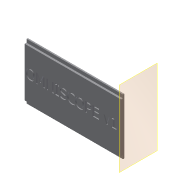
# Autodesk Inventor part: 01_Camera_Module_Lit
Saved by Autodesk Inventor 2019.4 (Build 234330000, 330)
## iProperties
Created: 2021-09-23
Part Number: 01_Camera_Module_Lit
Material: Generisch
Document SubType Name: Modeling
Designer: Muriel
Density: 1 g/cm^3
Appearance: Vorgabe
Mass: 2.33527 g
Surface Area: 32.2894 cm^2
Volume: 2.33527 cm^3
Author: Muriel
Autodesk Inventor part; units mm, degrees
ref_plane "YZ Plane" through (0, 0, 0) normal (1, 0, 0) x (0, 1, 0)
ref_plane "Arbeitsebene1" through (50, 3.7048, -4.525) normal (1, 0, 0) x (0, 0, -1)
sketch "Skizze1" plane through (50, 3.7048, -4.525) normal (1, 0, 0) x (0, 0, -1)
  line L0 (12.625, 1.4952) -> (9.775, 1.4952) projected
  line L1 (8.775, -0.2048) -> (8.475, -0.2048) projected
  line L2 (-3.525, -3.7048) -> (12.275, -3.7048) projected
  line L3 (13.275, -2.7048) -> (12.275, -3.7048) projected
  circle A0 centre (10.275, -2.1048) radius 0.95 projected
  circle A1 centre (-1.525, -2.1048) radius 0.95 projected
  line L4 (-2.525, 29.0952) -> (-2.525, 27.8724) projected
  line L5 (-1.025, 27.8724) -> (-2.525, 27.8724) projected
  line L6 (-1.025, 28.0952) -> (-1.025, 27.8724) projected
  line L7 (-0.025, 29.0952) -> (-1.025, 28.0952) projected
  line L8 (-0.025, 29.0952) -> (-2.525, 29.0952) projected
  line L9 (-4.525, 26.8952) -> (-2.825, 26.8952)
  line L10 (-2.825, 26.8952) -> (-2.825, 1.4952)
  line L11 (-2.825, 1.4952) -> (-4.525, 1.4952)
  line L12 (-4.525, 1.4952) -> (-4.525, 26.8952)
  line L13 (-2.825, 26.8952) -> (-3.525, 26.8952)
  line L14 (-3.525, 26.8952) -> (-3.525, 28.5952)
  line L15 (-3.525, 28.5952) -> (-2.825, 28.5952)
  line L16 (-2.825, 28.5952) -> (-2.825, 26.8952)
  line L17 (-2.825, 1.4952) -> (-3.525, 1.4952)
  line L18 (-3.525, 1.4952) -> (-3.525, -0.4048)
  line L19 (-3.525, -0.4048) -> (-2.825, -0.4048)
  line L20 (-2.825, -0.4048) -> (-2.825, 1.4952)
  line L21 (8.775, 28.5952) -> (8.475, 28.5952) projected
  line L22 (9.775, 26.8952) -> (9.775, 27.5952) projected
  line L23 (12.625, 26.8952) -> (9.775, 26.8952) projected
  line L24 (12.625, 1.4952) -> (12.625, 26.8952) projected
  line L25 (9.775, 1.4952) -> (9.775, 0.7952) projected
  line L26 (8.775, -0.2048) -> (9.775, 0.7952) projected
  line L27 (-3.525, -3.7048) -> (-4.525, -2.7048) projected
  line L28 (13.275, -2.7048) -> (13.275, 31.0952) projected
  line L29 (12.275, 32.0952) -> (13.275, 31.0952) projected
  line L30 (-3.525, 32.0952) -> (12.275, 32.0952) projected
  line L31 (-4.525, 31.0952) -> (-3.525, 32.0952) projected
  circle A2 centre (10.275, 30.4952) radius 0.95 projected
  circle A3 centre (-1.525, 30.4952) radius 0.95 projected
  line L32 (-3.6948, -0.7048) -> (-3.6948, 1.2952) projected
  line L33 (-4.525, 1.2952) -> (-4.525, -2.7048) projected
  line L34 (-4.525, 27.0952) -> (-4.525, 31.0952) projected
  line L35 (-3.6948, 27.0952) -> (-3.6948, 29.0952) projected
  line L36 (9.775, 27.5952) -> (8.775, 28.5952) projected
  line L37 (8.475, 29.0952) -> (8.475, 28.5952) projected
  line L38 (8.475, -0.2048) -> (8.475, -0.7048) projected
  line L39 (8.475, -0.7048) -> (-1.425, -0.7048) projected
  line L40 (-3.6948, 29.0952) -> (-2.425, 29.0952) projected
  line L41 (-1.425, 29.0952) -> (8.475, 29.0952) projected
  line L42 (-1.425, -0.7048) -> (-1.425, 0.2952) projected
  line L43 (-1.425, 0.2952) -> (-2.425, 0.2952) projected
  line L44 (-2.425, 0.2952) -> (-2.425, -0.7048) projected
  line L45 (-2.425, -0.7048) -> (-3.6948, -0.7048) projected
  line L46 (-3.6948, 1.2952) -> (-4.525, 1.2952) projected
  line L47 (-4.525, 27.0952) -> (-3.6948, 27.0952) projected
  line L48 (-2.425, 29.0952) -> (-2.425, 28.0952) projected
  line L49 (-2.425, 28.0952) -> (-1.425, 28.0952) projected
  line L50 (-1.425, 28.0952) -> (-1.425, 29.0952) projected
  point P0 (-4.525, -3.7048)
  point P1 (-3.525, 29.0952)
  point P2 (12.675, 25.9097)
  point P3 (12.675, 0.5181)
  point P4 (-4.525, -0.7048)
  point P5 (-4.525, 29.0952)
  point P6 (-1.525, -0.7048)
  point P7 (-2.525, 28.0952)
  point P8 (-1.525, 28.0952)
  point P9 (-1.525, 29.0952)
  point P10 (-2.525, -0.7048)
  constraints: 24 end point, 6 parallel, 3 horizontal, 3 perpendicular, 2 other
ref_plane "Arbeitsebene2" through (0, 5.25, -6.015) normal (-1, 0, 0) x (0, 0, 1)
ref_plane "Work Plane3" through (0, 1.51, -17.96) normal (1, 0, 0) x (0, 1, 0)
extrude "Extrusion1" add sketch "Skizze1" against normal up to surface (50 mm away) contours L9 L10 L11 L12 | L14 L15 L16 L9 | L11 L20 L19 L18
sketch "Skizze3" plane through (50, 5.2, 0) normal (0, 0, 1) x (1, 0, 0)
  line L0 (-49.4037, 15.6382) -> (-1.8416, 15.6382) construction
  line L1 (-1.8416, 15.6382) -> (-1.8416, 10.3786) construction
  line L2 (-1.8416, 10.3786) -> (-49.4037, 10.3786) construction
  line L3 (-49.4037, 10.3786) -> (-49.4037, 15.6382) construction
  spline S0 degree 2 poles (-45.3219, 14.9552) (-45.0356, 14.6198) (-44.7166, 13.6383) (-44.7166, 13.0084) knots 0 0 0 1 2 2 2
  spline S1 degree 2 poles (-44.7166, 13.0084) (-44.7166, 12.3949) (-45.0274, 11.4011) (-45.3219, 11.0657) knots 0 0 0 1 2 2 2
  spline S2 degree 2 poles (-45.3219, 11.0657) (-45.6327, 10.7139) (-46.4548, 10.3786) (-46.9497, 10.3786) knots 0 0 0 1 2 2 2
  spline S3 degree 2 poles (-46.9497, 10.3786) (-47.4609, 10.3786) (-48.2789, 10.7262) (-48.5775, 11.0657) knots 0 0 0 1 2 2 2
  spline S4 degree 2 poles (-48.5775, 11.0657) (-48.8679, 11.4011) (-49.1787, 12.3867) (-49.1787, 13.0084) knots 0 0 0 1 2 2 2
  spline S5 degree 2 poles (-49.1787, 13.0084) (-49.1787, 13.6423) (-48.8638, 14.6076) (-48.5734, 14.9552) knots 0 0 0 1 2 2 2
  spline S6 degree 2 poles (-48.5734, 14.9552) (-48.2789, 15.2906) (-47.4569, 15.6382) (-46.9497, 15.6382) knots 0 0 0 1 2 2 2
  spline S7 degree 2 poles (-46.9497, 15.6382) (-46.4344, 15.6382) (-45.6082, 15.2783) (-45.3219, 14.9552) knots 0 0 0 1 2 2 2
  spline S8 degree 2 poles (-45.416, 13.0084) (-45.416, 13.5074) (-45.6327, 14.2804) (-45.829, 14.534) knots 0 0 0 1 2 2 2
  spline S9 degree 2 poles (-45.829, 14.534) (-46.0295, 14.7957) (-46.5939, 15.0575) (-46.9456, 15.0575) knots 0 0 0 1 2 2 2
  spline S10 degree 2 poles (-46.9456, 15.0575) (-47.3096, 15.0575) (-47.8577, 14.8039) (-48.0663, 14.534) knots 0 0 0 1 2 2 2
  spline S11 degree 2 poles (-48.0663, 14.534) (-48.2667, 14.2763) (-48.4793, 13.4992) (-48.4793, 13.0084) knots 0 0 0 1 2 2 2
  spline S12 degree 2 poles (-48.4793, 13.0084) (-48.4793, 12.0145) (-47.645, 10.9593) (-46.9456, 10.9593) knots 0 0 0 1 2 2 2
  spline S13 degree 2 poles (-46.9456, 10.9593) (-46.2462, 10.9593) (-45.416, 12.0145) (-45.416, 13.0084) knots 0 0 0 1 2 2 2
  line L4 (-39.6532, 10.4849) -> (-40.324, 10.4849)
  line L5 (-40.324, 10.4849) -> (-40.324, 14.8325)
  line L6 (-40.324, 14.8325) -> (-41.6409, 11.8755)
  line L7 (-41.6409, 11.8755) -> (-42.0499, 11.8755)
  line L8 (-42.0499, 11.8755) -> (-43.3546, 14.8325)
  line L9 (-43.3546, 14.8325) -> (-43.3546, 10.4849)
  line L10 (-43.3546, 10.4849) -> (-43.9804, 10.4849)
  line L11 (-43.9804, 10.4849) -> (-43.9804, 15.5319)
  line L12 (-43.9804, 15.5319) -> (-43.0642, 15.5319)
  line L13 (-43.0642, 15.5319) -> (-41.8045, 12.7221)
  line L14 (-41.8045, 12.7221) -> (-40.5857, 15.5319)
  line L15 (-40.5857, 15.5319) -> (-39.6532, 15.5319)
  line L16 (-39.6532, 15.5319) -> (-39.6532, 10.4849)
  line L17 (-35.0193, 10.4849) -> (-35.7719, 10.4849)
  line L18 (-35.7719, 10.4849) -> (-38.005, 14.8366)
  line L19 (-38.005, 14.8366) -> (-38.005, 10.4849)
  line L20 (-38.005, 10.4849) -> (-38.6307, 10.4849)
  line L21 (-38.6307, 10.4849) -> (-38.6307, 15.5319)
  line L22 (-38.6307, 15.5319) -> (-37.6778, 15.5319)
  line L23 (-37.6778, 15.5319) -> (-35.6451, 11.536)
  line L24 (-35.6451, 11.536) -> (-35.6451, 15.5319)
  line L25 (-35.6451, 15.5319) -> (-35.0193, 15.5319)
  line L26 (-35.0193, 15.5319) -> (-35.0193, 10.4849)
  line L27 (-32.2381, 10.4849) -> (-34.1931, 10.4849)
  line L28 (-34.1931, 10.4849) -> (-34.1931, 11.0002)
  line L29 (-34.1931, 11.0002) -> (-33.551, 11.0002)
  line L30 (-33.551, 11.0002) -> (-33.551, 15.0166)
  line L31 (-33.551, 15.0166) -> (-34.1931, 15.0166)
  line L32 (-34.1931, 15.0166) -> (-34.1931, 15.5319)
  line L33 (-34.1931, 15.5319) -> (-32.2381, 15.5319)
  line L34 (-32.2381, 15.5319) -> (-32.2381, 15.0166)
  line L35 (-32.2381, 15.0166) -> (-32.8803, 15.0166)
  line L36 (-32.8803, 15.0166) -> (-32.8803, 11.0002)
  line L37 (-32.8803, 11.0002) -> (-32.2381, 11.0002)
  line L38 (-32.2381, 11.0002) -> (-32.2381, 10.4849)
  spline S14 degree 2 poles (-30.0009, 10.3949) (-30.549, 10.3949) (-31.3179, 10.624) (-31.6574, 10.7876) knots 0 0 0 1 2 2 2
  line L39 (-31.6574, 10.7876) -> (-31.6574, 11.6301)
  line L40 (-31.6574, 11.6301) -> (-31.6083, 11.6301)
  spline S15 degree 2 poles (-31.6083, 11.6301) (-31.277, 11.3193) (-30.4386, 10.9757) (-30.05, 10.9757) knots 0 0 0 1 2 2 2
  spline S16 degree 2 poles (-30.05, 10.9757) (-29.4938, 10.9757) (-28.9253, 11.4379) (-28.9253, 11.8182) knots 0 0 0 1 2 2 2
  spline S17 degree 2 poles (-28.9253, 11.8182) (-28.9253, 12.1209) (-29.2238, 12.4972) (-29.547, 12.5912) knots 0 0 0 1 2 2 2
  spline S18 degree 2 poles (-29.547, 12.5912) (-29.7801, 12.6567) (-30.1686, 12.7466) (-30.459, 12.8203) knots 0 0 0 1 2 2 2
  spline S19 degree 2 poles (-30.459, 12.8203) (-30.7208, 12.8898) (-31.1339, 13.0984) (-31.2934, 13.2661) knots 0 0 0 1 2 2 2
  spline S20 degree 2 poles (-31.2934, 13.2661) (-31.4488, 13.4338) (-31.6206, 13.8837) (-31.6206, 14.1781) knots 0 0 0 1 2 2 2
  spline S21 degree 2 poles (-31.6206, 14.1781) (-31.6206, 14.7916) (-30.6635, 15.6219) (-29.9232, 15.6219) knots 0 0 0 1 2 2 2
  spline S22 degree 2 poles (-29.9232, 15.6219) (-29.4979, 15.6219) (-28.7453, 15.4542) (-28.4222, 15.2947) knots 0 0 0 1 2 2 2
  line L41 (-28.4222, 15.2947) -> (-28.4222, 14.4931)
  line L42 (-28.4222, 14.4931) -> (-28.4713, 14.4931)
  spline S23 degree 2 poles (-28.4713, 14.4931) (-28.7126, 14.7139) (-29.4652, 15.0411) (-29.8782, 15.0411) knots 0 0 0 1 2 2 2
  spline S24 degree 2 poles (-29.8782, 15.0411) (-30.3445, 15.0411) (-30.9212, 14.6035) (-30.9212, 14.2477) knots 0 0 0 1 2 2 2
  spline S25 degree 2 poles (-30.9212, 14.2477) (-30.9212, 13.9286) (-30.5817, 13.5483) (-30.2627, 13.4624) knots 0 0 0 1 2 2 2
  spline S26 degree 2 poles (-30.2627, 13.4624) (-30.05, 13.4051) (-29.4324, 13.2579) (-29.2279, 13.1965) knots 0 0 0 1 2 2 2
  spline S27 degree 2 poles (-29.2279, 13.1965) (-28.7085, 13.037) (-28.2259, 12.3949) (-28.2259, 11.9246) knots 0 0 0 1 2 2 2
  spline S28 degree 2 poles (-28.2259, 11.9246) (-28.2259, 11.626) (-28.4672, 11.0534) (-28.684, 10.853) knots 0 0 0 1 2 2 2
  spline S29 degree 2 poles (-28.684, 10.853) (-28.9253, 10.6321) (-29.5388, 10.3949) (-30.0009, 10.3949) knots 0 0 0 1 2 2 2
  spline S30 degree 2 poles (-25.5715, 10.3949) (-26.0623, 10.3949) (-26.8926, 10.7262) (-27.1952, 11.0575) knots 0 0 0 1 2 2 2
  spline S31 degree 2 poles (-27.1952, 11.0575) (-27.4979, 11.3847) (-27.8292, 12.3663) (-27.8292, 13.0043) knots 0 0 0 1 2 2 2
  spline S32 degree 2 poles (-27.8292, 13.0043) (-27.8292, 13.6383) (-27.5061, 14.5789) (-27.1993, 14.9266) knots 0 0 0 1 2 2 2
  spline S33 degree 2 poles (-27.1993, 14.9266) (-26.8967, 15.2661) (-26.0705, 15.6219) (-25.5593, 15.6219) knots 0 0 0 1 2 2 2
  spline S34 degree 2 poles (-25.5593, 15.6219) (-25.3057, 15.6219) (-24.8599, 15.5483) (-24.6717, 15.491) knots 0 0 0 1 2 2 2
  spline S35 degree 2 poles (-24.6717, 15.491) (-24.5081, 15.4378) (-24.1687, 15.2865) (-24.001, 15.1965) knots 0 0 0 1 2 2 2
  line L43 (-24.001, 15.1965) -> (-24.001, 14.3867)
  line L44 (-24.001, 14.3867) -> (-24.0541, 14.3867)
  spline S36 degree 2 poles (-24.0541, 14.3867) (-24.1441, 14.4685) (-24.4222, 14.6976) (-24.6227, 14.808) knots 0 0 0 1 2 2 2
  spline S37 degree 2 poles (-24.6227, 14.808) (-24.8149, 14.9143) (-25.2689, 15.0493) (-25.5633, 15.0493) knots 0 0 0 1 2 2 2
  spline S38 degree 2 poles (-25.5633, 15.0493) (-25.8864, 15.0493) (-26.4631, 14.7834) (-26.6799, 14.5299) knots 0 0 0 1 2 2 2
  spline S39 degree 2 poles (-26.6799, 14.5299) (-26.8926, 14.2722) (-27.1298, 13.491) (-27.1298, 13.0043) knots 0 0 0 1 2 2 2
  spline S40 degree 2 poles (-27.1298, 13.0043) (-27.1298, 12.4849) (-26.8803, 11.7364) (-26.6635, 11.4788) knots 0 0 0 1 2 2 2
  spline S41 degree 2 poles (-26.6635, 11.4788) (-26.4509, 11.2293) (-25.8824, 10.9757) (-25.5633, 10.9757) knots 0 0 0 1 2 2 2
  spline S42 degree 2 poles (-25.5633, 10.9757) (-25.273, 10.9757) (-24.7781, 11.1188) (-24.5858, 11.2252) knots 0 0 0 1 2 2 2
  spline S43 degree 2 poles (-24.5858, 11.2252) (-24.4018, 11.3315) (-24.1278, 11.5524) (-24.0501, 11.6301) knots 0 0 0 1 2 2 2
  line L45 (-24.0501, 11.6301) -> (-24.001, 11.6301)
  line L46 (-24.001, 11.6301) -> (-24.001, 10.8285)
  spline S44 degree 2 poles (-24.001, 10.8285) (-24.1687, 10.7507) (-24.4631, 10.6076) (-24.6717, 10.5422) knots 0 0 0 1 2 2 2
  spline S45 degree 2 poles (-24.6717, 10.5422) (-24.8926, 10.4685) (-25.2689, 10.3949) (-25.5715, 10.3949) knots 0 0 0 1 2 2 2
  spline S46 degree 2 poles (-19.8047, 14.9552) (-19.5184, 14.6198) (-19.1994, 13.6383) (-19.1994, 13.0084) knots 0 0 0 1 2 2 2
  spline S47 degree 2 poles (-19.1994, 13.0084) (-19.1994, 12.3949) (-19.5102, 11.4011) (-19.8047, 11.0657) knots 0 0 0 1 2 2 2
  spline S48 degree 2 poles (-19.8047, 11.0657) (-20.1155, 10.7139) (-20.9376, 10.3786) (-21.4325, 10.3786) knots 0 0 0 1 2 2 2
  spline S49 degree 2 poles (-21.4325, 10.3786) (-21.9437, 10.3786) (-22.7617, 10.7262) (-23.0603, 11.0657) knots 0 0 0 1 2 2 2
  spline S50 degree 2 poles (-23.0603, 11.0657) (-23.3507, 11.4011) (-23.6615, 12.3867) (-23.6615, 13.0084) knots 0 0 0 1 2 2 2
  spline S51 degree 2 poles (-23.6615, 13.0084) (-23.6615, 13.6423) (-23.3466, 14.6076) (-23.0562, 14.9552) knots 0 0 0 1 2 2 2
  spline S52 degree 2 poles (-23.0562, 14.9552) (-22.7617, 15.2906) (-21.9396, 15.6382) (-21.4325, 15.6382) knots 0 0 0 1 2 2 2
  spline S53 degree 2 poles (-21.4325, 15.6382) (-20.9172, 15.6382) (-20.091, 15.2783) (-19.8047, 14.9552) knots 0 0 0 1 2 2 2
  spline S54 degree 2 poles (-19.8988, 13.0084) (-19.8988, 13.5074) (-20.1155, 14.2804) (-20.3118, 14.534) knots 0 0 0 1 2 2 2
  spline S55 degree 2 poles (-20.3118, 14.534) (-20.5123, 14.7957) (-21.0767, 15.0575) (-21.4284, 15.0575) knots 0 0 0 1 2 2 2
  spline S56 degree 2 poles (-21.4284, 15.0575) (-21.7924, 15.0575) (-22.3405, 14.8039) (-22.549, 14.534) knots 0 0 0 1 2 2 2
  spline S57 degree 2 poles (-22.549, 14.534) (-22.7495, 14.2763) (-22.9621, 13.4992) (-22.9621, 13.0084) knots 0 0 0 1 2 2 2
  spline S58 degree 2 poles (-22.9621, 13.0084) (-22.9621, 12.0145) (-22.1278, 10.9593) (-21.4284, 10.9593) knots 0 0 0 1 2 2 2
  spline S59 degree 2 poles (-21.4284, 10.9593) (-20.729, 10.9593) (-19.8988, 12.0145) (-19.8988, 13.0084) knots 0 0 0 1 2 2 2
  spline S60 degree 2 poles (-15.273, 14.0104) (-15.273, 13.6832) (-15.5062, 13.0943) (-15.7147, 12.8898) knots 0 0 0 1 2 2 2
  spline S61 degree 2 poles (-15.7147, 12.8898) (-15.9765, 12.6321) (-16.6841, 12.3663) (-17.2239, 12.3663) knots 0 0 0 1 2 2 2
  line L47 (-17.2239, 12.3663) -> (-17.7924, 12.3663)
  line L48 (-17.7924, 12.3663) -> (-17.7924, 10.4849)
  line L49 (-17.7924, 10.4849) -> (-18.4632, 10.4849)
  line L50 (-18.4632, 10.4849) -> (-18.4632, 15.5319)
  line L51 (-18.4632, 15.5319) -> (-17.1953, 15.5319)
  spline S62 degree 2 poles (-17.1953, 15.5319) (-16.7454, 15.5319) (-16.1156, 15.3847) (-15.8742, 15.217) knots 0 0 0 1 2 2 2
  spline S63 degree 2 poles (-15.8742, 15.217) (-15.592, 15.0247) (-15.273, 14.4317) (-15.273, 14.0104) knots 0 0 0 1 2 2 2
  spline S64 degree 2 poles (-15.9724, 13.99) (-15.9724, 14.2517) (-16.1524, 14.6362) (-16.3364, 14.7589) knots 0 0 0 1 2 2 2
  spline S65 degree 2 poles (-16.3364, 14.7589) (-16.4959, 14.8652) (-16.9213, 14.9511) (-17.2362, 14.9511) knots 0 0 0 1 2 2 2
  line L52 (-17.2362, 14.9511) -> (-17.7924, 14.9511)
  line L53 (-17.7924, 14.9511) -> (-17.7924, 12.9389)
  line L54 (-17.7924, 12.9389) -> (-17.3344, 12.9389)
  spline S66 degree 2 poles (-17.3344, 12.9389) (-16.9254, 12.9389) (-16.4223, 13.0698) (-16.2587, 13.2415) knots 0 0 0 1 2 2 2
  spline S67 degree 2 poles (-16.2587, 13.2415) (-16.1074, 13.3929) (-15.9724, 13.7487) (-15.9724, 13.99) knots 0 0 0 1 2 2 2
  line L55 (-14.635, 10.4849) -> (-14.635, 15.5319)
  line L56 (-14.635, 15.5319) -> (-11.4775, 15.5319)
  line L57 (-11.4775, 15.5319) -> (-11.4775, 14.9348)
  line L58 (-11.4775, 14.9348) -> (-13.9642, 14.9348)
  line L59 (-13.9642, 14.9348) -> (-13.9642, 13.5524)
  line L60 (-13.9642, 13.5524) -> (-11.6452, 13.5524)
  line L61 (-11.6452, 13.5524) -> (-11.6452, 12.9552)
  line L62 (-11.6452, 12.9552) -> (-13.9642, 12.9552)
  line L63 (-13.9642, 12.9552) -> (-13.9642, 11.082)
  line L64 (-13.9642, 11.082) -> (-11.4775, 11.082)
  line L65 (-11.4775, 11.082) -> (-11.4775, 10.4849)
  line L66 (-11.4775, 10.4849) -> (-14.635, 10.4849)
  line L67 (-5.6494, 14.2722) -> (-7.0768, 10.4849)
  line L68 (-7.0768, 10.4849) -> (-7.6494, 10.4849)
  line L69 (-7.6494, 10.4849) -> (-9.0645, 14.2722)
  line L70 (-9.0645, 14.2722) -> (-8.3733, 14.2722)
  line L71 (-8.3733, 14.2722) -> (-7.3385, 11.3561)
  line L72 (-7.3385, 11.3561) -> (-6.3119, 14.2722)
  line L73 (-6.3119, 14.2722) -> (-5.6494, 14.2722)
  line L74 (-2.4019, 10.4849) -> (-4.8641, 10.4849)
  line L75 (-4.8641, 10.4849) -> (-4.8641, 11.0002)
  line L76 (-4.8641, 11.0002) -> (-3.9479, 11.0002)
  line L77 (-3.9479, 11.0002) -> (-3.9479, 14.3826)
  line L78 (-3.9479, 14.3826) -> (-4.8641, 14.3826)
  line L79 (-4.8641, 14.3826) -> (-4.8641, 14.8448)
  spline S68 degree 2 poles (-4.8641, 14.8448) (-4.3447, 14.8448) (-3.8539, 15.1393) (-3.8212, 15.5483) knots 0 0 0 1 2 2 2
  line L80 (-3.8212, 15.5483) -> (-3.2976, 15.5483)
  line L81 (-3.2976, 15.5483) -> (-3.2976, 11.0002)
  line L82 (-3.2976, 11.0002) -> (-2.4019, 11.0002)
  line L83 (-2.4019, 11.0002) -> (-2.4019, 10.4849)
  point P0 (-50, -5.2)
  constraints: 2 other
extrude "Extrusion3" cut sketch "Skizze3" against normal blind 0.5
sketch "Sketch4" plane through (50, 3.3, -1.7) normal (0, 0, -1) x (-1, 0, 0)
  line L0 (50, 1.9) -> (50, 27.3) construction
  line L1 (0, 1.9) -> (50, 1.9) projected
  line L2 (0, 27.3) -> (0, 1.9) projected
  line L3 (0, 27.3) -> (50, 27.3) projected
  line L4 (2.4019, 12.9002) -> (2.4019, 12.3849) projected
  line L5 (2.4019, 12.3849) -> (4.8641, 12.3849) projected
  line L6 (4.8641, 12.3849) -> (4.8641, 12.9002) projected
  line L7 (4.8641, 12.9002) -> (3.9479, 12.9002) projected
  line L8 (3.9479, 12.9002) -> (3.9479, 16.2826) projected
  line L9 (3.9479, 16.2826) -> (4.8641, 16.2826) projected
  line L10 (4.8641, 16.2826) -> (4.8641, 16.7448) projected
  line L11 (3.8212, 17.4483) -> (3.2976, 17.4483) projected
  line L12 (3.2976, 17.4483) -> (3.2976, 12.9002) projected
  line L13 (3.2976, 12.9002) -> (2.4019, 12.9002) projected
  line L14 (11.4775, 12.3849) -> (14.635, 12.3849) construction
  line L15 (14.635, 12.3849) -> (14.635, 17.4319) construction
  line L16 (14.635, 17.4319) -> (11.4775, 17.4319) construction
  line L17 (11.4775, 17.4319) -> (11.4775, 16.8348) construction
  line L18 (11.4775, 16.8348) -> (13.9642, 16.8348) construction
  line L19 (13.9642, 16.8348) -> (13.9642, 15.4524) construction
  line L20 (13.9642, 15.4524) -> (11.6452, 15.4524) construction
  line L21 (11.6452, 15.4524) -> (11.6452, 14.8552) construction
  line L22 (11.6452, 14.8552) -> (13.9642, 14.8552) construction
  line L23 (13.9642, 14.8552) -> (13.9642, 12.982) construction
  line L24 (13.9642, 12.982) -> (11.4775, 12.982) construction
  line L25 (11.4775, 12.982) -> (11.4775, 12.3849) construction
  line L26 (17.2239, 14.2663) -> (17.7924, 14.2663) construction
  line L27 (17.7924, 14.2663) -> (17.7924, 12.3849) construction
  line L28 (17.7924, 12.3849) -> (18.4632, 12.3849) construction
  line L29 (18.4632, 12.3849) -> (18.4632, 17.4319) construction
  line L30 (18.4632, 17.4319) -> (17.1953, 17.4319) construction
  line L31 (31.6574, 12.6876) -> (31.6574, 13.5301) construction
  line L32 (31.6574, 13.5301) -> (31.6083, 13.5301) construction
  line L33 (28.4222, 17.1947) -> (28.4222, 16.3931) construction
  line L34 (28.4222, 16.3931) -> (28.4713, 16.3931) construction
  line L35 (35.0193, 17.4319) -> (35.0193, 12.3849) construction
  line L36 (35.0193, 12.3849) -> (35.7719, 12.3849) construction
  line L37 (35.7719, 12.3849) -> (38.005, 16.7366) construction
  line L38 (38.005, 16.7366) -> (38.005, 12.3849) construction
  line L39 (38.005, 12.3849) -> (38.6307, 12.3849) construction
  line L40 (38.6307, 12.3849) -> (38.6307, 17.4319) construction
  line L41 (38.6307, 17.4319) -> (37.6778, 17.4319) construction
  line L42 (37.6778, 17.4319) -> (35.6451, 13.436) construction
  line L43 (35.6451, 13.436) -> (35.6451, 17.4319) construction
  line L44 (35.6451, 17.4319) -> (35.0193, 17.4319) construction
  line L45 (39.6532, 17.4319) -> (39.6532, 12.3849) construction
  line L46 (39.6532, 12.3849) -> (40.324, 12.3849) construction
  line L47 (40.324, 12.3849) -> (40.324, 16.7325) construction
  line L48 (40.324, 16.7325) -> (41.6409, 13.7755) construction
  line L49 (41.6409, 13.7755) -> (42.0499, 13.7755) construction
  line L50 (42.0499, 13.7755) -> (43.3546, 16.7325) construction
  line L51 (43.3546, 16.7325) -> (43.3546, 12.3849) construction
  line L52 (43.3546, 12.3849) -> (43.9804, 12.3849) construction
  line L53 (43.9804, 12.3849) -> (43.9804, 17.4319) construction
  line L54 (43.9804, 17.4319) -> (43.0642, 17.4319) construction
  line L55 (43.0642, 17.4319) -> (41.8045, 14.6221) construction
  line L56 (41.8045, 14.6221) -> (40.5857, 17.4319) construction
  line L57 (40.5857, 17.4319) -> (39.6532, 17.4319) construction
  line L58 (32.2381, 12.9002) -> (32.2381, 12.3849) construction
  line L59 (32.2381, 12.3849) -> (34.1931, 12.3849) construction
  line L60 (34.1931, 12.3849) -> (34.1931, 12.9002) construction
  line L61 (34.1931, 12.9002) -> (33.551, 12.9002) construction
  line L62 (33.551, 12.9002) -> (33.551, 16.9166) construction
  line L63 (33.551, 16.9166) -> (34.1931, 16.9166) construction
  line L64 (34.1931, 16.9166) -> (34.1931, 17.4319) construction
  line L65 (34.1931, 17.4319) -> (32.2381, 17.4319) construction
  line L66 (32.2381, 17.4319) -> (32.2381, 16.9166) construction
  line L67 (32.2381, 16.9166) -> (32.8803, 16.9166) construction
  line L68 (32.8803, 16.9166) -> (32.8803, 12.9002) construction
  line L69 (32.8803, 12.9002) -> (32.2381, 12.9002) construction
  line L70 (24.001, 17.0965) -> (24.001, 16.2867) construction
  line L71 (24.001, 16.2867) -> (24.0541, 16.2867) construction
  line L72 (24.0501, 13.5301) -> (24.001, 13.5301) construction
  line L73 (24.001, 13.5301) -> (24.001, 12.7285) construction
  line L74 (6.3119, 16.1722) -> (5.6494, 16.1722) projected
  line L75 (5.6494, 16.1722) -> (7.0768, 12.3849) projected
  line L76 (7.0768, 12.3849) -> (7.6494, 12.3849) projected
  line L77 (7.6494, 12.3849) -> (9.0645, 16.1722) construction
  line L78 (9.0645, 16.1722) -> (8.3733, 16.1722) construction
  line L79 (8.3733, 16.1722) -> (7.3385, 13.2561) construction
  line L80 (7.3385, 13.2561) -> (6.3119, 16.1722) projected
  line L81 (13.8438, 5.0941) -> (50, 5.0941)
  line L82 (50, 5.0941) -> (50, 24.3341)
  line L83 (50, 24.3341) -> (13.8438, 24.3341)
  line L84 (13.8438, 24.3341) -> (13.8438, 5.0941)
  line L85 (13.8438, 5.0941) -> (50, 24.3341) construction
  line L86 (50, 5.0941) -> (13.8438, 24.3341) construction
  point P0 (50, -3.3)
  point P1 (15.8742, 17.117)
  point P2 (15.273, 15.9104)
  point P3 (15.7147, 14.7898)
  point P4 (21.4325, 17.5382)
  point P5 (19.8047, 16.8552)
  point P6 (19.1994, 14.9084)
  point P7 (19.8047, 12.9657)
  point P8 (21.4325, 12.2786)
  point P9 (23.0603, 12.9657)
  point P10 (23.6615, 14.9084)
  point P11 (23.0562, 16.8552)
  point P12 (28.684, 12.753)
  point P13 (30.0009, 12.2949)
  point P14 (30.05, 12.8757)
  point P15 (28.9253, 13.7182)
  point P16 (29.547, 14.4912)
  point P17 (30.459, 14.7203)
  point P18 (31.2934, 15.1661)
  point P19 (31.6206, 16.0781)
  point P20 (29.9232, 17.5219)
  point P21 (29.8782, 16.9411)
  point P22 (30.9212, 16.1477)
  point P23 (30.2627, 15.3624)
  point P24 (29.2279, 15.0965)
  point P25 (28.2259, 13.8246)
  point P26 (46.9497, 17.5382)
  point P27 (45.3219, 16.8552)
  point P28 (44.7166, 14.9084)
  point P29 (45.3219, 12.9657)
  point P30 (46.9497, 12.2786)
  point P31 (48.5775, 12.9657)
  point P32 (49.1787, 14.9084)
  point P33 (48.5734, 16.8552)
  point P34 (24.6717, 12.4422)
  point P35 (25.5715, 12.2949)
  point P36 (27.1952, 12.9575)
  point P37 (27.8292, 14.9043)
  point P38 (27.1993, 16.8266)
  point P39 (25.5593, 17.5219)
  point P40 (24.6717, 17.391)
  point P41 (24.6227, 16.708)
  point P42 (25.5633, 16.9493)
  point P43 (26.6799, 16.4299)
  point P44 (27.1298, 14.9043)
  point P45 (26.6635, 13.3788)
  point P46 (25.5633, 12.8757)
  point P47 (24.5858, 13.1252)
  point P48 (31.9219, 14.7141)
  constraints: 12 end point, 2 midpoint, 2 parallel, 1 horizontal, 1 perpendicular, 1 point on line, 53 other
extrude "Extrusion4" cut sketch "Sketch4" against normal blind 1
